Autodesk Inventor part; units mm, degrees
(part 2 of 2)
  circle A89 centre (160.02, 99.06) radius 0.508
  circle A90 centre (170.18, 99.06) radius 0.508
  circle A91 centre (177.8, 104.14) radius 0.508
  circle A92 centre (185.42, 99.06) radius 0.508
  circle A93 centre (195.58, 99.06) radius 0.508
  circle A94 centre (203.2, 104.14) radius 0.508
  circle A95 centre (210.82, 99.06) radius 0.508
  circle A96 centre (17.78, 124.46) radius 0.508
  circle A97 centre (25.4, 129.54) radius 0.508
  circle A98 centre (33.02, 124.46) radius 0.508
  circle A99 centre (43.18, 124.46) radius 0.508
  circle A100 centre (50.8, 129.54) radius 0.508
  circle A101 centre (58.42, 124.46) radius 0.508
  circle A102 centre (68.58, 124.46) radius 0.508
  circle A103 centre (76.2, 129.54) radius 0.508
  circle A104 centre (83.82, 124.46) radius 0.508
  circle A105 centre (93.98, 124.46) radius 0.508
  circle A106 centre (101.6, 129.54) radius 0.508
  circle A107 centre (109.22, 124.46) radius 0.508
  circle A108 centre (119.38, 124.46) radius 0.508
  circle A109 centre (127, 129.54) radius 0.508
  circle A110 centre (134.62, 124.46) radius 0.508
  circle A111 centre (144.78, 124.46) radius 0.508
  circle A112 centre (152.4, 129.54) radius 0.508
  circle A113 centre (160.02, 124.46) radius 0.508
  circle A114 centre (170.18, 124.46) radius 0.508
  circle A115 centre (177.8, 129.54) radius 0.508
  circle A116 centre (185.42, 124.46) radius 0.508
  circle A117 centre (195.58, 124.46) radius 0.508
  circle A118 centre (203.2, 129.54) radius 0.508
  circle A119 centre (210.82, 124.46) radius 0.508
  circle A120 centre (17.78, 149.86) radius 0.508
  circle A121 centre (25.4, 154.94) radius 0.508
  circle A122 centre (33.02, 149.86) radius 0.508
  circle A123 centre (43.18, 149.86) radius 0.508
  circle A124 centre (50.8, 154.94) radius 0.508
  circle A125 centre (58.42, 149.86) radius 0.508
  circle A126 centre (68.58, 149.86) radius 0.508
  circle A127 centre (76.2, 154.94) radius 0.508
  circle A128 centre (83.82, 149.86) radius 0.508
  circle A129 centre (93.98, 149.86) radius 0.508
  circle A130 centre (101.6, 154.94) radius 0.508
  circle A131 centre (109.22, 149.86) radius 0.508
  circle A132 centre (119.38, 149.86) radius 0.508
  circle A133 centre (127, 154.94) radius 0.508
  circle A134 centre (134.62, 149.86) radius 0.508
  circle A135 centre (144.78, 149.86) radius 0.508
  circle A136 centre (152.4, 154.94) radius 0.508
  circle A137 centre (160.02, 149.86) radius 0.508
  circle A138 centre (170.18, 149.86) radius 0.508
  circle A139 centre (177.8, 154.94) radius 0.508
  circle A140 centre (185.42, 149.86) radius 0.508
  circle A141 centre (195.58, 149.86) radius 0.508
  circle A142 centre (203.2, 154.94) radius 0.508
  circle A143 centre (210.82, 149.86) radius 0.508
  circle A144 centre (17.78, 175.26) radius 0.508
  circle A145 centre (25.4, 180.34) radius 0.508
  circle A146 centre (33.02, 175.26) radius 0.508
  circle A147 centre (43.18, 175.26) radius 0.508
  circle A148 centre (50.8, 180.34) radius 0.508
  circle A149 centre (58.42, 175.26) radius 0.508
  circle A150 centre (68.58, 175.26) radius 0.508
  circle A151 centre (76.2, 180.34) radius 0.508
  circle A152 centre (83.82, 175.26) radius 0.508
  circle A153 centre (93.98, 175.26) radius 0.508
  circle A154 centre (101.6, 180.34) radius 0.508
  circle A155 centre (109.22, 175.26) radius 0.508
  circle A156 centre (119.38, 175.26) radius 0.508
  circle A157 centre (127, 180.34) radius 0.508
  circle A158 centre (134.62, 175.26) radius 0.508
  circle A159 centre (144.78, 175.26) radius 0.508
  circle A160 centre (152.4, 180.34) radius 0.508
  circle A161 centre (160.02, 175.26) radius 0.508
  circle A162 centre (170.18, 175.26) radius 0.508
  circle A163 centre (177.8, 180.34) radius 0.508
  circle A164 centre (185.42, 175.26) radius 0.508
  circle A165 centre (195.58, 175.26) radius 0.508
  circle A166 centre (203.2, 180.34) radius 0.508
  circle A167 centre (210.82, 175.26) radius 0.508
  circle A168 centre (17.78, 200.66) radius 0.508
  circle A169 centre (25.4, 205.74) radius 0.508
  circle A170 centre (33.02, 200.66) radius 0.508
  circle A171 centre (43.18, 200.66) radius 0.508
  circle A172 centre (50.8, 205.74) radius 0.508
  circle A173 centre (58.42, 200.66) radius 0.508
  circle A174 centre (68.58, 200.66) radius 0.508
  circle A175 centre (76.2, 205.74) radius 0.508
  circle A176 centre (83.82, 200.66) radius 0.508
  circle A177 centre (93.98, 200.66) radius 0.508
  circle A178 centre (101.6, 205.74) radius 0.508
  circle A179 centre (109.22, 200.66) radius 0.508
  circle A180 centre (119.38, 200.66) radius 0.508
  circle A181 centre (127, 205.74) radius 0.508
  circle A182 centre (134.62, 200.66) radius 0.508
  circle A183 centre (144.78, 200.66) radius 0.508
  circle A184 centre (152.4, 205.74) radius 0.508
  circle A185 centre (160.02, 200.66) radius 0.508
  circle A186 centre (170.18, 200.66) radius 0.508
  circle A187 centre (177.8, 205.74) radius 0.508
  circle A188 centre (185.42, 200.66) radius 0.508
  circle A189 centre (195.58, 200.66) radius 0.508
  circle A190 centre (203.2, 205.74) radius 0.508
  circle A191 centre (210.82, 200.66) radius 0.508
  line L869 (228.6, 0) -> (228.6, 228.6) construction
  line L870 (228.6, 228.6) -> (194.6275, 228.6) construction
  line L871 (194.6275, 228.6) -> (194.6275, 213.614) construction
  line L872 (194.6275, 213.614) -> (228.6, 213.614) construction
  line L873 (228.6, 213.614) -> (228.6, 228.6) construction
  line L874 (194.6275, 213.614) -> (186.3725, 213.614)
  line L875 (186.3725, 213.614) -> (186.3725, 205.359)
  line L876 (186.3725, 205.359) -> (194.6275, 205.359)
  line L877 (194.6275, 205.359) -> (194.6275, 213.614)
  circle A192 centre (190.5, 205.359) radius 2.1336
  circle A193 centre (190.5, 205.359) radius 0.508
  line L878 (160.9725, 213.614) -> (160.9725, 205.359)
  line L879 (169.2275, 213.614) -> (160.9725, 213.614)
  line L880 (169.2275, 205.359) -> (169.2275, 213.614)
  line L881 (160.9725, 205.359) -> (169.2275, 205.359)
  circle A194 centre (165.1, 205.359) radius 2.1336
  circle A195 centre (165.1, 205.359) radius 0.508
  line L882 (135.5725, 213.614) -> (135.5725, 205.359)
  line L883 (143.8275, 213.614) -> (135.5725, 213.614)
  line L884 (143.8275, 205.359) -> (143.8275, 213.614)
  line L885 (135.5725, 205.359) -> (143.8275, 205.359)
  circle A196 centre (139.7, 205.359) radius 2.1336
  circle A197 centre (139.7, 205.359) radius 0.508
  line L886 (110.1725, 213.614) -> (110.1725, 205.359)
  line L887 (118.4275, 213.614) -> (110.1725, 213.614)
  line L888 (118.4275, 205.359) -> (118.4275, 213.614)
  line L889 (110.1725, 205.359) -> (118.4275, 205.359)
  circle A198 centre (114.3, 205.359) radius 2.1336
  circle A199 centre (114.3, 205.359) radius 0.508
  line L890 (84.7725, 213.614) -> (84.7725, 205.359)
  line L891 (93.0275, 213.614) -> (84.7725, 213.614)
  line L892 (93.0275, 205.359) -> (93.0275, 213.614)
  line L893 (84.7725, 205.359) -> (93.0275, 205.359)
  circle A200 centre (88.9, 205.359) radius 2.1336
  circle A201 centre (88.9, 205.359) radius 0.508
  line L894 (59.3725, 213.614) -> (59.3725, 205.359)
  line L895 (67.6275, 213.614) -> (59.3725, 213.614)
  line L896 (67.6275, 205.359) -> (67.6275, 213.614)
  line L897 (59.3725, 205.359) -> (67.6275, 205.359)
  circle A202 centre (63.5, 205.359) radius 2.1336
  circle A203 centre (63.5, 205.359) radius 0.508
  line L898 (33.9725, 213.614) -> (33.9725, 205.359)
  line L899 (42.2275, 213.614) -> (33.9725, 213.614)
  line L900 (42.2275, 205.359) -> (42.2275, 213.614)
  line L901 (33.9725, 205.359) -> (42.2275, 205.359)
  circle A204 centre (38.1, 205.359) radius 2.1336
  circle A205 centre (38.1, 205.359) radius 0.508
  line L902 (194.6275, 205.359) -> (194.6275, 199.263) construction
  line L903 (194.6275, 205.359) -> (200.7235, 205.359) construction
  line L904 (194.6275, 199.263) -> (192.0875, 199.263) construction
  line L905 (194.6275, 199.263) -> (197.1675, 199.263) construction
  line L906 (194.6275, 184.912) -> (186.3725, 184.912)
  line L907 (186.3725, 184.912) -> (186.3725, 193.167)
  line L908 (186.3725, 193.167) -> (194.6275, 193.167)
  line L909 (194.6275, 193.167) -> (194.6275, 184.912)
  circle A206 centre (190.5, 193.167) radius 2.1336
  circle A207 centre (190.5, 193.167) radius 0.508
  dimension "d6" = 82.55
  dimension "d7" = 12.7
  dimension "d8" = 63.5
  dimension "d9" = 2.54
  dimension "d10" = 17.78
  dimension "d11" = 2.54
  dimension "d14" = 22.86
  dimension "d21" = 25.4
  dimension "d26" = 0.635
  dimension "d27" = 0.762
  dimension "d28" = 1.27
  dimension "d29" = 2.286
  dimension "d32" = 5.08
  dimension "d37" = 0.635
  dimension "d38" = 0.762
  dimension "d39" = 2.286
  dimension "d42" = 5.08
  dimension "d49" = 25.4
  dimension "d52" = 22.86
  dimension "d55" = 17.78
  dimension "d56" = 22.86
  dimension "d57" = 1.016
  dimension "d58" = 15.24
  dimension "d60" = 1.016
  dimension "d61" = 5.08
  dimension "d62" = 1.016
  dimension "d65" = 25.4
  dimension "d68" = 25.4
  dimension "d71" = 33.9725
  dimension "d72" = 14.986
  dimension "d73" = 8.255
  dimension "d74" = 8.255
  dimension "d75" = 4.2672
  dimension "d76" = 1.016
  dimension "d79" = 25.4
  dimension "d84" = 6.096
  dimension "d86" = 2.54
  constraints: 1818 end point, 208 centre point, 21 horizontal, 20 parallel, 11 coincident, 11 perpendicular, 6 symmetric about line, 6 vertical, 3 equal length, 2 collinear, 2 midpoint, 2143 other
  measures "d6" distance of L1.end L2.end
  measures "d7" distance of L0.end L1.end
  measures "d8" distance of L6.end L5.end
  measures "d9" distance of L5.end L4.end
  measures "d10" distance of L10.end L9.end
  measures "d11" distance of L9.end L8.end
  measures "d14" distance of L6.end L12.start
  measures "d21" distance of L6.end L16.start
  measures "d26" distance of L87.end L88.end
  measures "d27" distance of L86.end L87.end
  measures "d28" distance of L91.end L92.end
  measures "d29" distance of L90.end L91.end
  measures "d32" distance of L90.end L94.start
  measures "d37" distance of L107.end L108.end
  measures "d38" distance of L106.end L107.end
  measures "d39" distance of L110.end L111.end
  measures "d42" distance of L107.end L114.start
  measures "d49" distance of L90.end L126.start
  measures "d52" distance of L90.end L350.start
  measures "d55" distance of L864.end L863.end
  measures "d56" distance of L863.end L862.end
  measures "d57" diameter of A0
  measures "d58" distance of L866.start L866.end
  measures "d60" diameter of A1
  measures "d61" distance of L868.start L868.end
  measures "d62" diameter of A2
  measures "d65" distance of L866.start A3.centre
  measures "d68" distance of L866.start A24.centre
  measures "d71" distance of L872.end L871.end
  measures "d72" distance of L871.end L870.end
  measures "d73" distance of L876.end L875.end
  measures "d74" distance of L875.end L874.end
  measures "d75" diameter of A192
  measures "d76" diameter of A193
  measures "d79" distance of L874.end L878.start
  measures "d84" distance of L876.end L902.end
  measures "d86" distance of L902.end L904.end
body "Solid1"
